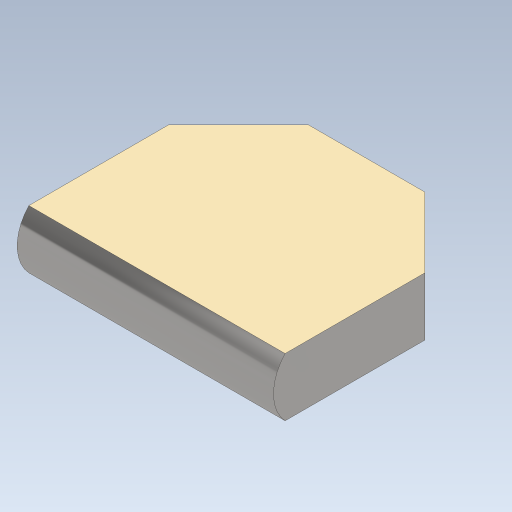
# Autodesk Inventor part: Pump-Motor-CW-Rotation:Vane
Saved by Autodesk Inventor 2024.2 (Build 282272000, 272)
## iProperties
Created: 2025-06-16
Material: Steel
Document SubType Name: Modeling
Density: 7.85 g/cm^3
Appearance: Steel - Polished
Designer: cw
Author: cw
Autodesk Inventor part; units mm, degrees
ref_plane "YZ Plane" through (0, 0, 0) normal (1, 0, 0) x (0, 1, 0)
ref_plane "XZ Plane" through (0, 0, 0) normal (0, 1, 0) x (-1, 0, 0)
ref_plane "XY Plane" through (0, 0, 0) normal (0, 0, 1) x (1, 0, 0)
sketch "Sketch1" plane through (0, 0, 0) normal (0, 0, 1) x (1, 0, 0)
  line L0 (-11, 0) -> (11, 0)
  line L1 (11, 0) -> (11, 19)
  line L2 (11, 19) -> (-11, 19)
  line L3 (-11, 19) -> (-11, 0)
  point P0 (0, 0)
  point P1 (0, 0)
  dimension "d0" = 22
  dimension "d1" = 19
  constraints: 8 end point, 2 parallel, 1 coincident, 1 horizontal, 1 midpoint, 1 perpendicular
  measures "d0" distance of L2.end L1.end
  measures "d1" distance of L1.end L0.end
extrude "Extrusion1" add sketch "Sketch1" along normal mid plane 5
chamfer "Chamfer1" distance 6 angle 45 2 edges at (-11, 19, 0) (11, 19, 0)
sketch "Sketch2" plane through (11, 0, 2.5) normal (1, 0, 0) x (0, 0, -1)
  line L0 (0, 0) -> (0, 13) projected
  line L1 (5, 13) -> (5, 0) projected
  arc A0 (0, 1) -> (5, 1) centre (2.5, 3.625) ccw
  line L2 (0, 0) -> (5, 0) projected
  point P0 (2.5, 0)
  point P1 (2.5, 0)
  dimension "d7" = 1
  constraints: 2 point on circle, 2 point on line, 1 centre point, 1 horizontal alignment, 1 tangent
  measures "d7" distance from line of A0.end L2
extrude "Extrusion2" cut sketch "Sketch2" against normal through all
body "Solid1"
